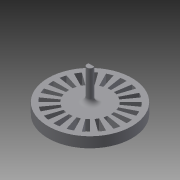
# Autodesk Inventor part: EncoderWheelAndPotInsert
Saved by Autodesk Inventor 2014 SP2 (Build 180246200, 246)
## iProperties
Created: 2014-10-31
Part Number: EncoderWheelAndPotInsert
Material: Generic
Document SubType Name: Modeling
Designer: Rebecca
Density: 1 g/cm^3
Appearance: Default
Author: Rebecca
Autodesk Inventor part; units mm, degrees
ref_plane "YZ Plane" through (0, 0, 0) normal (1, 0, 0) x (0, 1, 0)
ref_plane "XZ Plane" through (0, 0, 0) normal (0, 1, 0) x (-1, 0, 0)
ref_plane "XY Plane" through (0, 0, 0) normal (0, 0, 1) x (1, 0, 0)
sketch "Sketch1" plane through (0, 0, 0) normal (0, 1, 0) x (-1, 0, 0)
  circle A0 centre (0, 0) radius 25.4
  line L0 (12.7, 0) -> (22.225, 0)
  line L1 (12.5436, 1.9867) -> (21.9514, 3.4768)
  line L2 (0, 0) -> (22.225, 0) construction
  line L3 (0, 0) -> (22.225, 0) construction
  line L4 (0, 0) -> (22.225, 0) construction
  arc A1 (12.7, 0) -> (12.5436, 1.9867) centre (0, 0) ccw
  arc A2 (22.225, 0) -> (21.9514, 3.4768) centre (0, 0) ccw
  line L5 (12.0784, 3.9245) -> (21.1372, 6.8679)
  line L6 (11.3158, 5.7657) -> (19.8026, 10.0899)
  line L7 (0, 0) -> (21.1372, 6.8679) construction
  arc A3 (12.0784, 3.9245) -> (11.3158, 5.7657) centre (0, 0) ccw
  arc A4 (21.1372, 6.8679) -> (19.8026, 10.0899) centre (0, 0) ccw
  line L8 (10.2745, 7.4649) -> (17.9804, 13.0635)
  line L9 (8.9803, 8.9803) -> (15.7154, 15.7154)
  line L10 (0, 0) -> (17.9804, 13.0635) construction
  arc A5 (10.2745, 7.4649) -> (8.9803, 8.9803) centre (0, 0) ccw
  arc A6 (17.9804, 13.0635) -> (15.7154, 15.7154) centre (0, 0) ccw
  line L11 (7.4649, 10.2745) -> (13.0635, 17.9804)
  line L12 (5.7657, 11.3158) -> (10.0899, 19.8026)
  line L13 (0, 0) -> (13.0635, 17.9804) construction
  arc A7 (7.4649, 10.2745) -> (5.7657, 11.3158) centre (0, 0) ccw
  arc A8 (13.0635, 17.9804) -> (10.0899, 19.8026) centre (0, 0) ccw
  line L14 (3.9245, 12.0784) -> (6.8679, 21.1372)
  line L15 (1.9867, 12.5436) -> (3.4768, 21.9514)
  line L16 (0, 0) -> (6.8679, 21.1372) construction
  arc A9 (3.9245, 12.0784) -> (1.9867, 12.5436) centre (0, 0) ccw
  arc A10 (6.8679, 21.1372) -> (3.4768, 21.9514) centre (0, 0) ccw
  line L17 (0, 12.7) -> (0, 22.225)
  line L18 (-1.9867, 12.5436) -> (-3.4768, 21.9514)
  line L19 (0, 0) -> (0, 22.225) construction
  arc A11 (0, 12.7) -> (-1.9867, 12.5436) centre (0, 0) ccw
  arc A12 (0, 22.225) -> (-3.4768, 21.9514) centre (0, 0) ccw
  line L20 (-3.9245, 12.0784) -> (-6.8679, 21.1372)
  line L21 (-5.7657, 11.3158) -> (-10.0899, 19.8026)
  line L22 (0, 0) -> (-6.8679, 21.1372) construction
  arc A13 (-3.9245, 12.0784) -> (-5.7657, 11.3158) centre (0, 0) ccw
  arc A14 (-6.8679, 21.1372) -> (-10.0899, 19.8026) centre (0, 0) ccw
  line L23 (-7.4649, 10.2745) -> (-13.0635, 17.9804)
  line L24 (-8.9803, 8.9803) -> (-15.7154, 15.7154)
  line L25 (0, 0) -> (-13.0635, 17.9804) construction
  arc A15 (-7.4649, 10.2745) -> (-8.9803, 8.9803) centre (0, 0) ccw
  arc A16 (-13.0635, 17.9804) -> (-15.7154, 15.7154) centre (0, 0) ccw
  line L26 (-10.2745, 7.4649) -> (-17.9804, 13.0635)
  line L27 (-11.3158, 5.7657) -> (-19.8026, 10.0899)
  line L28 (0, 0) -> (-17.9804, 13.0635) construction
  arc A17 (-10.2745, 7.4649) -> (-11.3158, 5.7657) centre (0, 0) ccw
  arc A18 (-17.9804, 13.0635) -> (-19.8026, 10.0899) centre (0, 0) ccw
  line L29 (-12.0784, 3.9245) -> (-21.1372, 6.8679)
  line L30 (-12.5436, 1.9867) -> (-21.9514, 3.4768)
  line L31 (0, 0) -> (-21.1372, 6.8679) construction
  arc A19 (-12.0784, 3.9245) -> (-12.5436, 1.9867) centre (0, 0) ccw
  arc A20 (-21.1372, 6.8679) -> (-21.9514, 3.4768) centre (0, 0) ccw
  line L32 (-12.7, 0) -> (-22.225, 0)
  line L33 (-12.5436, -1.9867) -> (-21.9514, -3.4768)
  line L34 (0, 0) -> (-22.225, 0) construction
  arc A21 (-12.7, 0) -> (-12.5436, -1.9867) centre (0, 0) ccw
  arc A22 (-22.225, 0) -> (-21.9514, -3.4768) centre (0, 0) ccw
  line L35 (-12.0784, -3.9245) -> (-21.1372, -6.8679)
  line L36 (-11.3158, -5.7657) -> (-19.8026, -10.0899)
  line L37 (0, 0) -> (-21.1372, -6.8679) construction
  arc A23 (-12.0784, -3.9245) -> (-11.3158, -5.7657) centre (0, 0) ccw
  arc A24 (-21.1372, -6.8679) -> (-19.8026, -10.0899) centre (0, 0) ccw
  line L38 (-10.2745, -7.4649) -> (-17.9804, -13.0635)
  line L39 (-8.9803, -8.9803) -> (-15.7154, -15.7154)
  line L40 (0, 0) -> (-17.9804, -13.0635) construction
  arc A25 (-10.2745, -7.4649) -> (-8.9803, -8.9803) centre (0, 0) ccw
  arc A26 (-17.9804, -13.0635) -> (-15.7154, -15.7154) centre (0, 0) ccw
  line L41 (-7.4649, -10.2745) -> (-13.0635, -17.9804)
  line L42 (-5.7657, -11.3158) -> (-10.0899, -19.8026)
  line L43 (0, 0) -> (-13.0635, -17.9804) construction
  arc A27 (-7.4649, -10.2745) -> (-5.7657, -11.3158) centre (0, 0) ccw
  arc A28 (-13.0635, -17.9804) -> (-10.0899, -19.8026) centre (0, 0) ccw
  line L44 (-3.9245, -12.0784) -> (-6.8679, -21.1372)
  line L45 (-1.9867, -12.5436) -> (-3.4768, -21.9514)
  line L46 (0, 0) -> (-6.8679, -21.1372) construction
  arc A29 (-3.9245, -12.0784) -> (-1.9867, -12.5436) centre (0, 0) ccw
  arc A30 (-6.8679, -21.1372) -> (-3.4768, -21.9514) centre (0, 0) ccw
  line L47 (0, -12.7) -> (0, -22.225)
  line L48 (1.9867, -12.5436) -> (3.4768, -21.9514)
  line L49 (0, 0) -> (0, -22.225) construction
  arc A31 (0, -12.7) -> (1.9867, -12.5436) centre (0, 0) ccw
  arc A32 (0, -22.225) -> (3.4768, -21.9514) centre (0, 0) ccw
  line L50 (3.9245, -12.0784) -> (6.8679, -21.1372)
  line L51 (5.7657, -11.3158) -> (10.0899, -19.8026)
  line L52 (0, 0) -> (6.8679, -21.1372) construction
  arc A33 (3.9245, -12.0784) -> (5.7657, -11.3158) centre (0, 0) ccw
  arc A34 (6.8679, -21.1372) -> (10.0899, -19.8026) centre (0, 0) ccw
  line L53 (7.4649, -10.2745) -> (13.0635, -17.9804)
  line L54 (8.9803, -8.9803) -> (15.7154, -15.7154)
  line L55 (0, 0) -> (13.0635, -17.9804) construction
  arc A35 (7.4649, -10.2745) -> (8.9803, -8.9803) centre (0, 0) ccw
  arc A36 (13.0635, -17.9804) -> (15.7154, -15.7154) centre (0, 0) ccw
  line L56 (10.2745, -7.4649) -> (17.9804, -13.0635)
  line L57 (11.3158, -5.7657) -> (19.8026, -10.0899)
  line L58 (0, 0) -> (17.9804, -13.0635) construction
  arc A37 (10.2745, -7.4649) -> (11.3158, -5.7657) centre (0, 0) ccw
  arc A38 (17.9804, -13.0635) -> (19.8026, -10.0899) centre (0, 0) ccw
  line L59 (12.0784, -3.9245) -> (21.1372, -6.8679)
  line L60 (12.5436, -1.9867) -> (21.9514, -3.4768)
  line L61 (0, 0) -> (21.1372, -6.8679) construction
  arc A39 (12.0784, -3.9245) -> (12.5436, -1.9867) centre (0, 0) ccw
  arc A40 (21.1372, -6.8679) -> (21.9514, -3.4768) centre (0, 0) ccw
  dimension "d0" = 50.8
  dimension "d3" = 9
  dimension "d9" = 360
  constraints: 124 end point, 120 point on circle, 41 centre point, 24 coincident, 4 horizontal, 299 other
  measures "d0" diameter of A0
  measures "d3" angle of L2 L1
extrude "Extrusion1" add sketch "Sketch1" along normal blind 6.35
sketch "Sketch2" plane through (0, 6.35, 0) normal (0, 1, 0) x (1, 0, 0)
  arc A0 (-22.225, 0) -> (-21.9514, -3.4768) centre (0, 0) ccw projected
  arc A1 (-1.6848, 0.889) -> (1.6848, 0.889) centre (0, 0) ccw
  line L0 (1.6848, 0.889) -> (-1.6848, 0.889)
  dimension "d23" = 3.81
  constraints: 2 end point, 2 point on circle, 1 centre point, 1 coincident
  measures "d23" diameter of A1
extrude "Extrusion2" add sketch "Sketch2" along normal blind 19.05
sketch "Sketch3" plane through (0, 0, 0) normal (0, -1, 0) x (1, 0, 0)
  circle A0 centre (0, 0) radius 25.4 projected
  arc A1 (1.1581, -0.9906) -> (-1.1581, -0.9906) centre (0, 0) ccw
  line L0 (-1.1581, -0.9906) -> (1.1581, -0.9906)
  dimension "d19" = 3.048
  constraints: 2 end point, 2 point on circle, 1 centre point, 1 coincident
  measures "d19" diameter of A1
extrude "Extrusion3" cut sketch "Sketch3" against normal blind 3.175 contours L0 A1
fillet "Fillet3" radius 3.175 2 edges at (0, 6.35, -0.889) (0, 6.35, 1.905)
body "Solid1"
